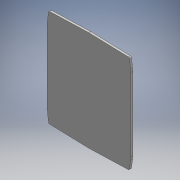
# Autodesk Inventor part: End
Saved by Autodesk Inventor 2016 (Build 200138000, 138)
## iProperties
Created: 2016-04-18
Part Number: End
Material: Generic
Document SubType Name: Modeling
Designer: Jarrett
Density: 1 g/cm^3
Appearance: Default
Author: Jarrett
Autodesk Inventor part; units mm, degrees
ref_plane "YZ Plane" through (0, 0, 0) normal (1, 0, 0) x (0, 1, 0)
ref_plane "XZ Plane" through (0, 0, 0) normal (0, 1, 0) x (-1, 0, 0)
ref_plane "XY Plane" through (0, 0, 0) normal (0, 0, 1) x (1, 0, 0)
sketch "Sketch1" plane through (0, 0, 0) normal (0, 1, 0) x (-1, 0, 0)
  line L0 (0, 0) -> (36.25, 0) construction
  line L1 (36.25, 0) -> (36.25, 31.6619)
  line L2 (36.0718, 34.3261) -> (35.1129, 41.4603)
  line L3 (34.1532, 42.3266) -> (0, 43.4)
  line L4 (0, 43.4) -> (0, 0) construction
  arc A0 (35.1129, 41.4603) -> (34.1532, 42.3266) centre (34.1218, 41.3271) ccw
  arc A1 (36.25, 31.6619) -> (36.0718, 34.3261) centre (16.25, 31.6619) ccw
  line L5 (36.25, 0) -> (36.25, -31.6619)
  line L6 (36.0718, -34.3261) -> (35.1129, -41.4603)
  line L7 (34.1532, -42.3266) -> (0, -43.4)
  arc A2 (34.1532, -42.3266) -> (35.1129, -41.4603) centre (34.1218, -41.3271) ccw
  arc A3 (36.0718, -34.3261) -> (36.25, -31.6619) centre (16.25, -31.6619) ccw
  line L8 (-36.25, 0) -> (-36.25, 31.6619)
  line L9 (-36.0718, 34.3261) -> (-35.1129, 41.4603)
  line L10 (-34.1532, 42.3266) -> (0, 43.4)
  arc A4 (-34.1532, 42.3266) -> (-35.1129, 41.4603) centre (-34.1218, 41.3271) ccw
  arc A5 (-36.0718, 34.3261) -> (-36.25, 31.6619) centre (-16.25, 31.6619) ccw
  line L11 (-36.0718, -34.3261) -> (-35.1129, -41.4603)
  arc A6 (-35.1129, -41.4603) -> (-34.1532, -42.3266) centre (-34.1218, -41.3271) ccw
  arc A7 (-36.25, -31.6619) -> (-36.0718, -34.3261) centre (-16.25, -31.6619) ccw
  line L12 (-36.25, 0) -> (-36.25, -31.6619)
  line L13 (-34.1532, -42.3266) -> (0, -43.4)
  point P0 (36.25, 33)
  point P1 (35, 42.3)
  point P2 (36.25, -33)
  point P3 (35, -42.3)
  point P4 (-36.25, 33)
  point P5 (-35, 42.3)
  point P6 (-36.25, -33)
  point P7 (-35, -42.3)
  dimension "d2" = 36.25
  dimension "d3" = 43.4
  dimension "d6" = 33
  dimension "d7" = 9.3
  dimension "d8" = 35
  dimension "d9" = 1
  dimension "d10" = 20
  constraints: 28 end point, 26 symmetric about line, 16 point on circle, 16 point on line, 8 centre point, 4 tangent, 2 horizontal, 2 vertical, 1 parallel, 6 other
  measures "d2" distance of L0.start L0.end
  measures "d3" distance of L3.end L0.start
  measures "d6" distance from line of point (36.25, 33) L0
  measures "d7" vertical distance of point (36.25, 33) point (35, 42.3)
  measures "d8" horizontal distance of point (35, 42.3) L3.end
  measures "d9" radius of A0
  measures "d10" radius of A1
extrude "Extrusion1" add sketch "Sketch1" along normal blind 1.7
body "Solid1"
